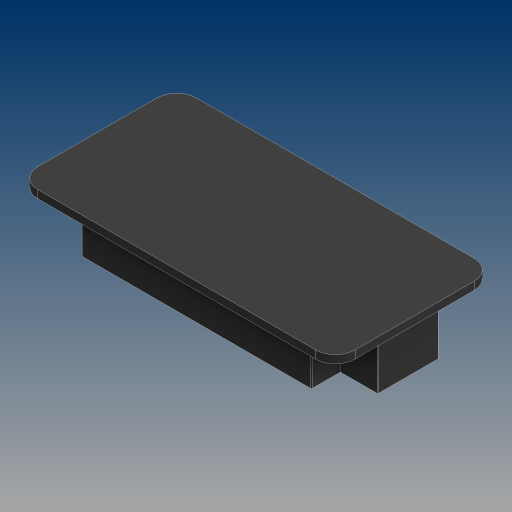
# Autodesk Inventor part: ELEV_011_EXTRUENDCAP
Saved by Autodesk Inventor 2024.3 (Build 283343000, 343)
## iProperties
Created: 2024-11-26
Part Number: ELEV_011_EXTRUENDCAP
Material: Rubber
Document SubType Name: Modeling
Designer: Kenji
Density: 0.93 g/cm^3
Appearance: Rubber - Black
Author: Kenji
Autodesk Inventor part; units mm, degrees
ref_plane "YZ Plane" through (0, 0, 0) normal (1, 0, 0) x (0, 1, 0)
ref_plane "XZ Plane" through (0, 0, 0) normal (0, 1, 0) x (-1, 0, 0)
ref_plane "XY Plane" through (0, 0, 0) normal (0, 0, 1) x (1, 0, 0)
sketch "Sketch1" plane through (0, 0, 0) normal (0, 1, 0) x (-1, 0, 0)
  line L0 (0, -0.127) -> (0, -9.652)
  line L1 (0.127, -9.779) -> (5.9944, -9.779)
  line L2 (5.9944, -9.779) -> (5.9944, -14.2875)
  line L3 (6.1214, -14.4145) -> (42.6466, -14.4145)
  line L4 (42.7736, -14.2875) -> (42.7736, -9.779)
  line L5 (42.7736, -9.779) -> (48.641, -9.779)
  line L6 (48.768, -9.652) -> (48.768, -0.127)
  line L7 (48.641, 0) -> (42.7736, 0)
  line L8 (42.7736, 0) -> (42.7736, 4.5085)
  line L9 (42.6466, 4.6355) -> (6.1214, 4.6355)
  line L10 (5.9944, 4.5085) -> (5.9944, 0)
  line L11 (0.127, 0) -> (5.9944, 0)
  arc A0 (48.768, -0.127) -> (48.641, 0) centre (48.641, -0.127) ccw
  arc A1 (48.641, -9.779) -> (48.768, -9.652) centre (48.641, -9.652) ccw
  arc A2 (42.6466, -14.4145) -> (42.7736, -14.2875) centre (42.6466, -14.2875) ccw
  arc A3 (5.9944, -14.2875) -> (6.1214, -14.4145) centre (6.1214, -14.2875) ccw
  arc A4 (0, -9.652) -> (0.127, -9.779) centre (0.127, -9.652) ccw
  arc A5 (0.127, 0) -> (0, -0.127) centre (0.127, -0.127) ccw
  arc A6 (6.1214, 4.6355) -> (5.9944, 4.5085) centre (6.1214, 4.5085) ccw
  arc A7 (42.7736, 4.5085) -> (42.6466, 4.6355) centre (42.6466, 4.5085) ccw
  point P0 (0, 0)
  point P1 (42.7736, 4.6355)
  point P2 (5.9944, 4.6355)
  dimension "d0" = 48.768
  dimension "d1" = 19.05
  dimension "d2" = 9.779
  dimension "d3" = 36.7792
  dimension "d4" = 0.127
  constraints: 24 end point, 16 point on circle, 16 tangent, 11 point on line, 9 perpendicular, 8 centre point, 7 equal radius, 3 collinear, 1 horizontal
  measures "d0" distance between parallel lines of L0 L6
  measures "d1" distance between parallel lines of L3 L9
  measures "d2" distance between parallel lines of L5 L7
  measures "d3" distance between parallel lines of L10 L8
  measures "d4" radius of A0
extrude "Extrusion1" add sketch "Sketch1" along normal blind 7.62
sketch "Sketch2" plane through (0, 7.62, 0) normal (0, 1, 0) x (1, 0, 0)
  line L0 (0, 0.127) -> (0, 9.652) projected
  arc A0 (0, 9.652) -> (-0.127, 9.779) centre (-0.127, 9.652) ccw projected
  line L1 (-0.127, 9.779) -> (-5.9944, 9.779) projected
  line L2 (-5.9944, 9.779) -> (-5.9944, 14.2875) projected
  arc A1 (-5.9944, 14.2875) -> (-6.1214, 14.4145) centre (-6.1214, 14.2875) ccw projected
  line L3 (-6.1214, 14.4145) -> (-42.6466, 14.4145) projected
  arc A2 (-42.6466, 14.4145) -> (-42.7736, 14.2875) centre (-42.6466, 14.2875) ccw projected
  line L4 (-42.7736, 14.2875) -> (-42.7736, 9.779) projected
  line L5 (-42.7736, 9.779) -> (-48.641, 9.779) projected
  arc A3 (-48.641, 9.779) -> (-48.768, 9.652) centre (-48.641, 9.652) ccw projected
  line L6 (-48.768, 9.652) -> (-48.768, 0.127) projected
  arc A4 (-48.768, 0.127) -> (-48.641, 0) centre (-48.641, 0.127) ccw projected
  line L7 (-48.641, 0) -> (-42.7736, 0) projected
  line L8 (-42.7736, 0) -> (-42.7736, -4.5085) projected
  arc A5 (-42.7736, -4.5085) -> (-42.6466, -4.6355) centre (-42.6466, -4.5085) ccw projected
  line L9 (-42.6466, -4.6355) -> (-6.1214, -4.6355) projected
  arc A6 (-6.1214, -4.6355) -> (-5.9944, -4.5085) centre (-6.1214, -4.5085) ccw projected
  line L10 (-5.9944, -4.5085) -> (-5.9944, 0) projected
  line L11 (-5.9944, 0) -> (-0.127, 0) projected
  arc A7 (-0.127, 0) -> (0, 0.127) centre (-0.127, 0.127) ccw projected
  line L12 (-46.609, 17.5895) -> (-2.159, 17.5895)
  line L13 (1.016, 14.4145) -> (1.016, -4.6355)
  line L14 (-2.159, -7.8105) -> (-46.609, -7.8105)
  line L15 (-49.784, -4.6355) -> (-49.784, 14.4145)
  arc A8 (-46.609, 17.5895) -> (-49.784, 14.4145) centre (-46.609, 14.4145) ccw
  arc A9 (1.016, 14.4145) -> (-2.159, 17.5895) centre (-2.159, 14.4145) ccw
  arc A10 (-2.159, -7.8105) -> (1.016, -4.6355) centre (-2.159, -4.6355) ccw
  arc A11 (-49.784, -4.6355) -> (-46.609, -7.8105) centre (-46.609, -4.6355) ccw
  dimension "d10" = 50.8
  dimension "d11" = 25.4
  dimension "d12" = 48.768
  dimension "d13" = 1.016
  dimension "d14" = 19.05
  dimension "d15" = 3.175
  dimension "d16" = 3.175
  constraints: 8 end point, 8 point on circle, 8 tangent, 4 centre point, 3 equal radius, 2 parallel, 1 horizontal, 1 perpendicular
  measures "d10" distance between parallel lines of L15 L13
  measures "d11" distance between parallel lines of L14 L12
  measures "d12" distance between parallel lines of L0 L6
  measures "d13" distance between parallel lines of L15 L6
  measures "d14" distance between parallel lines of L9 L3
  measures "d15" distance between parallel lines of L3 L12
  measures "d16" radius of A8
extrude "Extrusion3" add sketch "Sketch2" along normal blind 1.27 contours A7 L11 L10 A6 L9 A5 L8 L7 A4 L6 A3 L5 L4 A2 L3 A1 L2 L1 A0 L0 | L12 A9 L13 A10 L14 A11 L15 A8
body "Solid1"
